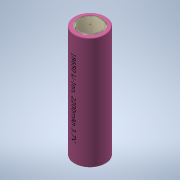
# Autodesk Inventor part: 18650
Saved by Autodesk Inventor 2022 (Build 260153070, 153G)
## iProperties
Created: 2016-01-10
Part Number: 18650
Material: Generic
Document SubType Name: Modeling
Designer: Kostic
Density: 1 g/cm^3
Appearance: Default
GlobalPropertyList: <PropertyList/>
Author: Kostic
Autodesk Inventor part; units mm, degrees
ref_plane "YZ Plane" through (0, 0, 0) normal (1, 0, 0) x (0, 1, 0)
ref_plane "XY Plane" through (0, 0, 0) normal (0, 0, 1) x (1, 0, 0)
sketch "Sketch1" plane through (0, 0, 0) normal (0, 0, 1) x (1, 0, 0)
  circle A0 centre (0, 0) radius 9
  dimension "d0" = 18
  constraints: 1 centre point, 1 coincident
  measures "d0" diameter of A0
extrude "Extrusion1" add sketch "Sketch1" along normal blind 64.7
sketch "Sketch2" plane through (0, 0, 64.7) normal (0, 0, 1) x (1, 0, 0)
  circle A0 centre (0, 0) radius 6
  dimension "d3" = 12
  constraints: 1 centre point, 1 coincident
  measures "d3" diameter of A0
extrude "Extrusion2" add sketch "Sketch2" along normal blind 0.1
sketch "Sketch3" plane through (0, 0, 0) normal (0, 0, -1) x (-1, 0, 0)
  circle A0 centre (0, 0) radius 7
  dimension "d6" = 14
  constraints: 1 centre point, 1 coincident
  measures "d6" diameter of A0
extrude "Extrusion3" cut sketch "Sketch3" against normal blind 0.1
fillet "Fillet1" radius 0.5 2 edges at (-9, 0, 64.7) (-9, 0, 0)
sketch "Sketch4" plane through (0, 0, 64.7) normal (0, 0, 1) x (1, 0, 0)
  circle A0 centre (0, 0) radius 7
  circle A1 centre (0, 0) radius 6
  dimension "d10" = 14
  dimension "d11" = 12
  constraints: 2 centre point, 2 coincident
  measures "d10" diameter of A0
  measures "d11" diameter of A1
extrude "Extrusion4" cut sketch "Sketch4" against normal blind 0.6
fillet "Fillet2" radius 0.5 2 edges at (-7, 0, 64.1) (-6, 0, 64.1)
fillet "Fillet3" radius 0.1 1 edges at (-6, 0, 64.8)
ref_plane "Work Plane1" through (0, -9, 0) normal (0, -1, 0) x (1, 0, 0)
sketch "Sketch5" plane through (0, -9, 0) normal (0, -1, 0) x (1, 0, 0)
  line L0 (0.9968, 55) -> (0.9968, -8.1341) construction
  line L1 (0.9968, -8.1341) -> (-3.5299, -8.1341) construction
  line L2 (-3.5299, -8.1341) -> (-3.5299, 55) construction
  line L3 (-3.5299, 55) -> (0.9968, 55) construction
  line L4 (8.5, 0) -> (-8.5, 0) projected
  line L5 (-1.6564, 53.376) -> (-1.6564, 54.6151)
  line L6 (-1.6564, 54.6151) -> (-1.397, 54.6151)
  line L7 (-1.397, 54.6151) -> (-1.397, 54.154)
  line L8 (-1.397, 54.154) -> (0.3052, 54.154)
  line L9 (0.3052, 54.154) -> (0.3052, 54.6151)
  line L10 (0.3052, 54.6151) -> (0.5378, 54.6151)
  spline S0 degree 2 poles (0.5378, 54.6151) (0.5378, 54.3537) (0.686, 54.1067) (0.8919, 54.0902) knots 0 0 0 1 2 2 2
  line L11 (0.8919, 54.0902) -> (0.8919, 53.8267)
  line L12 (0.8919, 53.8267) -> (-1.397, 53.8267)
  line L13 (-1.397, 53.8267) -> (-1.397, 53.376)
  line L14 (-1.397, 53.376) -> (-1.6564, 53.376)
  spline S1 degree 2 poles (-1.714, 52.141) (-1.714, 52.3303) (-1.6008, 52.6411) (-1.4958, 52.7502) knots 0 0 0 1 2 2 2
  spline S2 degree 2 poles (-1.4958, 52.7502) (-1.3929, 52.8573) (-1.113, 52.9684) (-0.9545, 52.9684) knots 0 0 0 1 2 2 2
  spline S3 degree 2 poles (-0.9545, 52.9684) (-0.7486, 52.9684) (-0.4028, 52.7482) (-0.2999, 52.5382) knots 0 0 0 1 2 2 2
  line L15 (-0.2999, 52.5382) -> (-0.2896, 52.5382)
  spline S4 degree 2 poles (-0.2896, 52.5382) (-0.1805, 52.7255) (0.0788, 52.9067) (0.2723, 52.9067) knots 0 0 0 1 2 2 2
  spline S5 degree 2 poles (0.2723, 52.9067) (0.5584, 52.9067) (0.9413, 52.4744) (0.9413, 52.141) knots 0 0 0 1 2 2 2
  spline S6 degree 2 poles (0.9413, 52.141) (0.9413, 51.7952) (0.579, 51.3773) (0.295, 51.3773) knots 0 0 0 1 2 2 2
  spline S7 degree 2 poles (0.295, 51.3773) (0.1241, 51.3773) (-0.2093, 51.577) (-0.304, 51.7643) knots 0 0 0 1 2 2 2
  line L16 (-0.304, 51.7643) -> (-0.3143, 51.7643)
  spline S8 degree 2 poles (-0.3143, 51.7643) (-0.4172, 51.542) (-0.7136, 51.3135) (-0.9483, 51.3135) knots 0 0 0 1 2 2 2
  spline S9 degree 2 poles (-0.9483, 51.3135) (-1.2735, 51.3135) (-1.714, 51.7869) (-1.714, 52.141) knots 0 0 0 1 2 2 2
  spline S10 degree 2 poles (-0.9812, 51.6634) (-0.8248, 51.6634) (-0.6395, 51.7869) (-0.5449, 51.9619) knots 0 0 0 1 2 2 2
  spline S11 degree 2 poles (-0.5449, 51.9619) (-0.5119, 52.0195) (-0.4358, 52.213) (-0.3864, 52.3344) knots 0 0 0 1 2 2 2
  spline S12 degree 2 poles (-0.3864, 52.3344) (-0.479, 52.4744) (-0.7548, 52.6247) (-0.9298, 52.6247) knots 0 0 0 1 2 2 2
  spline S13 degree 2 poles (-0.9298, 52.6247) (-1.1603, 52.6247) (-1.4608, 52.3468) (-1.4608, 52.1368) knots 0 0 0 1 2 2 2
  spline S14 degree 2 poles (-1.4608, 52.1368) (-1.4608, 51.9228) (-1.2035, 51.6634) (-0.9812, 51.6634) knots 0 0 0 1 2 2 2
  spline S15 degree 2 poles (0.2908, 51.7108) (0.4617, 51.7108) (0.6902, 51.9392) (0.6902, 52.143) knots 0 0 0 1 2 2 2
  spline S16 degree 2 poles (0.6902, 52.143) (0.6902, 52.3283) (0.4864, 52.565) (0.3114, 52.565) knots 0 0 0 1 2 2 2
  spline S17 degree 2 poles (0.3114, 52.565) (0.1859, 52.565) (0.0109, 52.4435) (-0.0591, 52.3221) knots 0 0 0 1 2 2 2
  spline S18 degree 2 poles (-0.0591, 52.3221) (-0.0879, 52.2706) (-0.1888, 52.0524) (-0.2176, 51.9639) knots 0 0 0 1 2 2 2
  spline S19 degree 2 poles (-0.2176, 51.9639) (-0.1044, 51.8157) (0.1365, 51.7108) (0.2908, 51.7108) knots 0 0 0 1 2 2 2
  spline S20 degree 2 poles (-0.833, 49.3972) (-1.0286, 49.3972) (-1.36, 49.5269) (-1.4711, 49.6359) knots 0 0 0 1 2 2 2
  spline S21 degree 2 poles (-1.4711, 49.6359) (-1.5884, 49.7492) (-1.7099, 50.0332) (-1.7099, 50.2041) knots 0 0 0 1 2 2 2
  spline S22 degree 2 poles (-1.7099, 50.2041) (-1.7099, 50.3749) (-1.5946, 50.6569) (-1.4793, 50.7639) knots 0 0 0 1 2 2 2
  spline S23 degree 2 poles (-1.4793, 50.7639) (-1.3414, 50.8957) (-0.8783, 51.0439) (-0.5407, 51.0439) knots 0 0 0 1 2 2 2
  spline S24 degree 2 poles (-0.5407, 51.0439) (-0.2093, 51.0439) (0.3238, 50.908) (0.5214, 50.766) knots 0 0 0 1 2 2 2
  spline S25 degree 2 poles (0.5214, 50.766) (0.7149, 50.6281) (0.931, 50.1917) (0.931, 49.9056) knots 0 0 0 1 2 2 2
  spline S26 degree 2 poles (0.931, 49.9056) (0.931, 49.8212) (0.9145, 49.673) (0.896, 49.6174) knots 0 0 0 1 2 2 2
  line L17 (0.896, 49.6174) -> (0.5687, 49.6174)
  line L18 (0.5687, 49.6174) -> (0.5687, 49.6318)
  spline S27 degree 2 poles (0.5687, 49.6318) (0.5934, 49.6792) (0.6366, 49.8521) (0.6366, 49.9509) knots 0 0 0 1 2 2 2
  spline S28 degree 2 poles (0.6366, 49.9509) (0.6366, 50.2679) (0.2085, 50.6569) (-0.2114, 50.6939) knots 0 0 0 1 2 2 2
  spline S29 degree 2 poles (-0.2114, 50.6939) (-0.127, 50.5725) (-0.0344, 50.3173) (-0.0344, 50.1649) knots 0 0 0 1 2 2 2
  spline S30 degree 2 poles (-0.0344, 50.1649) (-0.0344, 50.0167) (-0.0941, 49.7944) (-0.1846, 49.673) knots 0 0 0 1 2 2 2
  spline S31 degree 2 poles (-0.1846, 49.673) (-0.2896, 49.533) (-0.6148, 49.3972) (-0.833, 49.3972) knots 0 0 0 1 2 2 2
  spline S32 degree 2 poles (-0.8474, 49.743) (-0.691, 49.743) (-0.479, 49.8253) (-0.4049, 49.9159) knots 0 0 0 1 2 2 2
  spline S33 degree 2 poles (-0.4049, 49.9159) (-0.3514, 49.9838) (-0.3164, 50.1526) (-0.3164, 50.2411) knots 0 0 0 1 2 2 2
  spline S34 degree 2 poles (-0.3164, 50.2411) (-0.3164, 50.3605) (-0.3884, 50.5848) (-0.4563, 50.6939) knots 0 0 0 1 2 2 2
  spline S35 degree 2 poles (-0.4563, 50.6939) (-0.4934, 50.696) (-0.5634, 50.7001) (-0.6169, 50.7001) knots 0 0 0 1 2 2 2
  spline S36 degree 2 poles (-0.6169, 50.7001) (-0.8804, 50.7001) (-1.2035, 50.5972) (-1.2879, 50.519) knots 0 0 0 1 2 2 2
  spline S37 degree 2 poles (-1.2879, 50.519) (-1.3682, 50.4469) (-1.432, 50.2905) (-1.432, 50.202) knots 0 0 0 1 2 2 2
  spline S38 degree 2 poles (-1.432, 50.202) (-1.432, 49.9962) (-1.1397, 49.743) (-0.8474, 49.743) knots 0 0 0 1 2 2 2
  spline S39 degree 2 poles (-0.8495, 47.557) (-1.0327, 47.557) (-1.3455, 47.6743) (-1.4608, 47.7814) knots 0 0 0 1 2 2 2
  spline S40 degree 2 poles (-1.4608, 47.7814) (-1.5761, 47.8884) (-1.7099, 48.2075) (-1.7099, 48.4051) knots 0 0 0 1 2 2 2
  spline S41 degree 2 poles (-1.7099, 48.4051) (-1.7099, 48.5862) (-1.6296, 48.9402) (-1.5658, 49.0699) knots 0 0 0 1 2 2 2
  line L19 (-1.5658, 49.0699) -> (-1.2056, 49.0699)
  line L20 (-1.2056, 49.0699) -> (-1.2056, 49.0452)
  spline S42 degree 2 poles (-1.2056, 49.0452) (-1.2344, 49.0061) (-1.3085, 48.86) (-1.3414, 48.7714) knots 0 0 0 1 2 2 2
  spline S43 degree 2 poles (-1.3414, 48.7714) (-1.3764, 48.6706) (-1.4155, 48.5039) (-1.4155, 48.3989) knots 0 0 0 1 2 2 2
  spline S44 degree 2 poles (-1.4155, 48.3989) (-1.4155, 48.296) (-1.3414, 48.1025) (-1.2612, 48.0325) knots 0 0 0 1 2 2 2
  spline S45 degree 2 poles (-1.2612, 48.0325) (-1.185, 47.9687) (-0.9833, 47.9028) (-0.8474, 47.9028) knots 0 0 0 1 2 2 2
  spline S46 degree 2 poles (-0.8474, 47.9028) (-0.7116, 47.9028) (-0.5387, 47.9769) (-0.481, 48.0469) knots 0 0 0 1 2 2 2
  spline S47 degree 2 poles (-0.481, 48.0469) (-0.4172, 48.1189) (-0.3637, 48.333) (-0.3637, 48.4627) knots 0 0 0 1 2 2 2
  spline S48 degree 2 poles (-0.3637, 48.4627) (-0.3637, 48.6027) (-0.4069, 48.8805) (-0.4255, 48.9649) knots 0 0 0 1 2 2 2
  line L21 (-0.4255, 48.9649) -> (0.8836, 48.9649)
  line L22 (0.8836, 48.9649) -> (0.8836, 47.5714)
  line L23 (0.8836, 47.5714) -> (0.5852, 47.5714)
  line L24 (0.5852, 47.5714) -> (0.5852, 48.6376)
  line L25 (0.5852, 48.6376) -> (-0.092, 48.6376)
  spline S49 degree 2 poles (-0.092, 48.6376) (-0.0838, 48.5759) (-0.0776, 48.4565) (-0.0776, 48.4071) knots 0 0 0 1 2 2 2
  spline S50 degree 2 poles (-0.0776, 48.4071) (-0.0776, 48.2116) (-0.1414, 47.9419) (-0.2361, 47.8184) knots 0 0 0 1 2 2 2
  spline S51 degree 2 poles (-0.2361, 47.8184) (-0.3308, 47.6929) (-0.619, 47.557) (-0.8495, 47.557) knots 0 0 0 1 2 2 2
  spline S52 degree 2 poles (-0.3864, 45.6098) (-1.0697, 45.6098) (-1.7099, 46.0071) (-1.7099, 46.4208) knots 0 0 0 1 2 2 2
  spline S53 degree 2 poles (-1.7099, 46.4208) (-1.7099, 46.8407) (-1.0574, 47.2339) (-0.3884, 47.2339) knots 0 0 0 1 2 2 2
  spline S54 degree 2 poles (-0.3884, 47.2339) (0.2991, 47.2339) (0.9351, 46.8366) (0.9351, 46.4208) knots 0 0 0 1 2 2 2
  spline S55 degree 2 poles (0.9351, 46.4208) (0.9351, 46.003) (0.2764, 45.6098) (-0.3864, 45.6098) knots 0 0 0 1 2 2 2
  spline S56 degree 2 poles (-1.1603, 46.0462) (-1.0347, 45.9968) (-0.6478, 45.9556) (-0.3864, 45.9556) knots 0 0 0 1 2 2 2
  spline S57 degree 2 poles (-0.3864, 45.9556) (-0.1249, 45.9556) (0.26, 45.9968) (0.3896, 46.0482) knots 0 0 0 1 2 2 2
  spline S58 degree 2 poles (0.3896, 46.0482) (0.5193, 46.0997) (0.6531, 46.2788) (0.6531, 46.4208) knots 0 0 0 1 2 2 2
  spline S59 degree 2 poles (0.6531, 46.4208) (0.6531, 46.5628) (0.5193, 46.746) (0.3855, 46.7995) knots 0 0 0 1 2 2 2
  spline S60 degree 2 poles (0.3855, 46.7995) (0.2558, 46.851) (-0.1394, 46.8881) (-0.3884, 46.8881) knots 0 0 0 1 2 2 2
  spline S61 degree 2 poles (-0.3884, 46.8881) (-0.656, 46.8881) (-1.0142, 46.8551) (-1.1541, 46.8016) knots 0 0 0 1 2 2 2
  spline S62 degree 2 poles (-1.1541, 46.8016) (-1.2859, 46.7522) (-1.4279, 46.569) (-1.4279, 46.4208) knots 0 0 0 1 2 2 2
  spline S63 degree 2 poles (-1.4279, 46.4208) (-1.4279, 46.2808) (-1.2941, 46.0976) (-1.1603, 46.0462) knots 0 0 0 1 2 2 2
  line L26 (-1.6564, 42.6499) -> (-1.6564, 44.1216)
  line L27 (-1.6564, 44.1216) -> (0.8836, 44.1216)
  line L28 (0.8836, 44.1216) -> (0.8836, 43.7841)
  line L29 (0.8836, 43.7841) -> (-1.3558, 43.7841)
  line L30 (-1.3558, 43.7841) -> (-1.3558, 42.6499)
  line L31 (-1.3558, 42.6499) -> (-1.6564, 42.6499)
  line L32 (-1.6564, 42.0818) -> (-1.6564, 42.4029)
  line L33 (-1.6564, 42.4029) -> (0.2497, 42.4029)
  line L34 (0.2497, 42.4029) -> (0.2497, 42.0818)
  line L35 (0.2497, 42.0818) -> (-1.6564, 42.0818)
  line L36 (0.5667, 42.0592) -> (0.5667, 42.4235)
  line L37 (0.5667, 42.4235) -> (0.9001, 42.4235)
  line L38 (0.9001, 42.4235) -> (0.9001, 42.0592)
  line L39 (0.9001, 42.0592) -> (0.5667, 42.0592)
  line L40 (-0.6992, 40.7274) -> (-0.6992, 41.6887)
  line L41 (-0.6992, 41.6887) -> (-0.3905, 41.6887)
  line L42 (-0.3905, 41.6887) -> (-0.3905, 40.7274)
  line L43 (-0.3905, 40.7274) -> (-0.6992, 40.7274)
  line L44 (-1.6564, 39.4327) -> (-1.6564, 40.4166)
  line L45 (-1.6564, 40.4166) -> (-1.397, 40.4166)
  line L46 (-1.397, 40.4166) -> (-1.397, 40.0935)
  line L47 (-1.397, 40.0935) -> (0.6243, 40.0935)
  line L48 (0.6243, 40.0935) -> (0.6243, 40.4166)
  line L49 (0.6243, 40.4166) -> (0.8836, 40.4166)
  line L50 (0.8836, 40.4166) -> (0.8836, 39.4327)
  line L51 (0.8836, 39.4327) -> (0.6243, 39.4327)
  line L52 (0.6243, 39.4327) -> (0.6243, 39.7559)
  line L53 (0.6243, 39.7559) -> (-1.397, 39.7559)
  line L54 (-1.397, 39.7559) -> (-1.397, 39.4327)
  line L55 (-1.397, 39.4327) -> (-1.6564, 39.4327)
  spline S64 degree 2 poles (-0.7033, 37.4732) (-1.185, 37.4732) (-1.7099, 37.9363) (-1.7099, 38.3233) knots 0 0 0 1 2 2 2
  spline S65 degree 2 poles (-1.7099, 38.3233) (-1.7099, 38.7205) (-1.1685, 39.1754) (-0.7033, 39.1754) knots 0 0 0 1 2 2 2
  spline S66 degree 2 poles (-0.7033, 39.1754) (-0.2258, 39.1754) (0.3032, 38.7061) (0.3032, 38.3233) knots 0 0 0 1 2 2 2
  spline S67 degree 2 poles (0.3032, 38.3233) (0.3032, 37.9363) (-0.2238, 37.4732) (-0.7033, 37.4732) knots 0 0 0 1 2 2 2
  spline S68 degree 2 poles (-0.7033, 37.8046) (-0.3328, 37.8046) (0.0274, 38.0742) (0.0274, 38.3233) knots 0 0 0 1 2 2 2
  spline S69 degree 2 poles (0.0274, 38.3233) (0.0274, 38.5723) (-0.3328, 38.844) (-0.7033, 38.844) knots 0 0 0 1 2 2 2
  spline S70 degree 2 poles (-0.7033, 38.844) (-1.0636, 38.844) (-1.4341, 38.5723) (-1.4341, 38.3233) knots 0 0 0 1 2 2 2
  spline S71 degree 2 poles (-1.4341, 38.3233) (-1.4341, 38.0763) (-1.0697, 37.8046) (-0.7033, 37.8046) knots 0 0 0 1 2 2 2
  line L56 (-1.6564, 35.6474) -> (-1.6564, 35.9685)
  line L57 (-1.6564, 35.9685) -> (-0.5696, 35.9685)
  spline S72 degree 2 poles (-0.5696, 35.9685) (-0.4378, 35.9685) (-0.2114, 35.9932) (-0.1435, 36.0303) knots 0 0 0 1 2 2 2
  spline S73 degree 2 poles (-0.1435, 36.0303) (-0.0714, 36.0694) (-0.0014, 36.2094) (-0.0014, 36.3287) knots 0 0 0 1 2 2 2
  spline S74 degree 2 poles (-0.0014, 36.3287) (-0.0014, 36.4481) (-0.1291, 36.7013) (-0.232, 36.8227) knots 0 0 0 1 2 2 2
  line L58 (-0.232, 36.8227) -> (-1.6564, 36.8227)
  line L59 (-1.6564, 36.8227) -> (-1.6564, 37.1438)
  line L60 (-1.6564, 37.1438) -> (0.2497, 37.1438)
  line L61 (0.2497, 37.1438) -> (0.2497, 36.8227)
  line L62 (0.2497, 36.8227) -> (0.0377, 36.8227)
  spline S75 degree 2 poles (0.0377, 36.8227) (0.1673, 36.6787) (0.3032, 36.4008) (0.3032, 36.2443) knots 0 0 0 1 2 2 2
  spline S76 degree 2 poles (0.3032, 36.2443) (0.3032, 35.9644) (-0.0673, 35.6474) (-0.4193, 35.6474) knots 0 0 0 1 2 2 2
  line L63 (-0.4193, 35.6474) -> (-1.6564, 35.6474)
  line L64 (-1.1706, 34.5771) -> (-2.2883, 35.0546)
  line L65 (-2.2883, 35.0546) -> (-2.2883, 35.3037)
  line L66 (-2.2883, 35.3037) -> (-1.1706, 35.0032)
  line L67 (-1.1706, 35.0032) -> (-1.1706, 34.5771)
  line L68 (-1.6564, 31.5287) -> (-1.6564, 33.0951)
  line L69 (-1.6564, 33.0951) -> (-1.2961, 33.0951)
  spline S77 degree 2 poles (-1.2961, 33.0951) (-1.1377, 32.9263) (-0.8433, 32.6258) (-0.6848, 32.4817) knots 0 0 0 1 2 2 2
  spline S78 degree 2 poles (-0.6848, 32.4817) (-0.3658, 32.1915) (0.0171, 31.9794) (0.2209, 31.9794) knots 0 0 0 1 2 2 2
  spline S79 degree 2 poles (0.2209, 31.9794) (0.3279, 31.9794) (0.4884, 32.0453) (0.5399, 32.105) knots 0 0 0 1 2 2 2
  spline S80 degree 2 poles (0.5399, 32.105) (0.5914, 32.1647) (0.6428, 32.3211) (0.6428, 32.4158) knots 0 0 0 1 2 2 2
  spline S81 degree 2 poles (0.6428, 32.4158) (0.6428, 32.5064) (0.5975, 32.6916) (0.5625, 32.776) knots 0 0 0 1 2 2 2
  spline S82 degree 2 poles (0.5625, 32.776) (0.5337, 32.8481) (0.4514, 32.9819) (0.4226, 33.023) knots 0 0 0 1 2 2 2
  line L70 (0.4226, 33.023) -> (0.4226, 33.0416)
  line L71 (0.4226, 33.0416) -> (0.7848, 33.0416)
  spline S83 degree 2 poles (0.7848, 33.0416) (0.8363, 32.9366) (0.9372, 32.5599) (0.9372, 32.3911) knots 0 0 0 1 2 2 2
  spline S84 degree 2 poles (0.9372, 32.3911) (0.9372, 32.035) (0.5605, 31.6336) (0.2394, 31.6336) knots 0 0 0 1 2 2 2
  spline S85 degree 2 poles (0.2394, 31.6336) (0.0891, 31.6336) (-0.162, 31.7036) (-0.269, 31.7654) knots 0 0 0 1 2 2 2
  spline S86 degree 2 poles (-0.269, 31.7654) (-0.3802, 31.8271) (-0.5984, 32.0062) (-0.7033, 32.105) knots 0 0 0 1 2 2 2
  spline S87 degree 2 poles (-0.7033, 32.105) (-0.8783, 32.2656) (-1.2529, 32.6587) (-1.362, 32.776) knots 0 0 0 1 2 2 2
  line L72 (-1.362, 32.776) -> (-1.362, 31.5287)
  line L73 (-1.362, 31.5287) -> (-1.6564, 31.5287)
  line L74 (-1.6564, 29.6226) -> (-1.6564, 31.189)
  line L75 (-1.6564, 31.189) -> (-1.2961, 31.189)
  spline S88 degree 2 poles (-1.2961, 31.189) (-1.1377, 31.0203) (-0.8433, 30.7197) (-0.6848, 30.5757) knots 0 0 0 1 2 2 2
  spline S89 degree 2 poles (-0.6848, 30.5757) (-0.3658, 30.2854) (0.0171, 30.0734) (0.2209, 30.0734) knots 0 0 0 1 2 2 2
  spline S90 degree 2 poles (0.2209, 30.0734) (0.3279, 30.0734) (0.4884, 30.1393) (0.5399, 30.199) knots 0 0 0 1 2 2 2
  spline S91 degree 2 poles (0.5399, 30.199) (0.5914, 30.2587) (0.6428, 30.4151) (0.6428, 30.5098) knots 0 0 0 1 2 2 2
  spline S92 degree 2 poles (0.6428, 30.5098) (0.6428, 30.6004) (0.5975, 30.7856) (0.5625, 30.87) knots 0 0 0 1 2 2 2
  spline S93 degree 2 poles (0.5625, 30.87) (0.5337, 30.942) (0.4514, 31.0758) (0.4226, 31.117) knots 0 0 0 1 2 2 2
  line L76 (0.4226, 31.117) -> (0.4226, 31.1355)
  line L77 (0.4226, 31.1355) -> (0.7848, 31.1355)
  spline S94 degree 2 poles (0.7848, 31.1355) (0.8363, 31.0306) (0.9372, 30.6539) (0.9372, 30.4851) knots 0 0 0 1 2 2 2
  spline S95 degree 2 poles (0.9372, 30.4851) (0.9372, 30.129) (0.5605, 29.7276) (0.2394, 29.7276) knots 0 0 0 1 2 2 2
  spline S96 degree 2 poles (0.2394, 29.7276) (0.0891, 29.7276) (-0.162, 29.7976) (-0.269, 29.8594) knots 0 0 0 1 2 2 2
  spline S97 degree 2 poles (-0.269, 29.8594) (-0.3802, 29.9211) (-0.5984, 30.1002) (-0.7033, 30.199) knots 0 0 0 1 2 2 2
  spline S98 degree 2 poles (-0.7033, 30.199) (-0.8783, 30.3595) (-1.2529, 30.7527) (-1.362, 30.87) knots 0 0 0 1 2 2 2
  line L78 (-1.362, 30.87) -> (-1.362, 29.6226)
  line L79 (-1.362, 29.6226) -> (-1.6564, 29.6226)
  spline S99 degree 2 poles (-0.3864, 27.7022) (-1.0697, 27.7022) (-1.7099, 28.0995) (-1.7099, 28.5132) knots 0 0 0 1 2 2 2
  spline S100 degree 2 poles (-1.7099, 28.5132) (-1.7099, 28.9331) (-1.0574, 29.3262) (-0.3884, 29.3262) knots 0 0 0 1 2 2 2
  spline S101 degree 2 poles (-0.3884, 29.3262) (0.2991, 29.3262) (0.9351, 28.929) (0.9351, 28.5132) knots 0 0 0 1 2 2 2
  spline S102 degree 2 poles (0.9351, 28.5132) (0.9351, 28.0953) (0.2764, 27.7022) (-0.3864, 27.7022) knots 0 0 0 1 2 2 2
  spline S103 degree 2 poles (-1.1603, 28.1386) (-1.0347, 28.0892) (-0.6478, 28.048) (-0.3864, 28.048) knots 0 0 0 1 2 2 2
  spline S104 degree 2 poles (-0.3864, 28.048) (-0.1249, 28.048) (0.26, 28.0892) (0.3896, 28.1406) knots 0 0 0 1 2 2 2
  spline S105 degree 2 poles (0.3896, 28.1406) (0.5193, 28.1921) (0.6531, 28.3712) (0.6531, 28.5132) knots 0 0 0 1 2 2 2
  spline S106 degree 2 poles (0.6531, 28.5132) (0.6531, 28.6552) (0.5193, 28.8384) (0.3855, 28.8919) knots 0 0 0 1 2 2 2
  spline S107 degree 2 poles (0.3855, 28.8919) (0.2558, 28.9434) (-0.1394, 28.9804) (-0.3884, 28.9804) knots 0 0 0 1 2 2 2
  spline S108 degree 2 poles (-0.3884, 28.9804) (-0.656, 28.9804) (-1.0142, 28.9475) (-1.1541, 28.894) knots 0 0 0 1 2 2 2
  spline S109 degree 2 poles (-1.1541, 28.894) (-1.2859, 28.8446) (-1.4279, 28.6614) (-1.4279, 28.5132) knots 0 0 0 1 2 2 2
  spline S110 degree 2 poles (-1.4279, 28.5132) (-1.4279, 28.3732) (-1.2941, 28.19) (-1.1603, 28.1386) knots 0 0 0 1 2 2 2
  spline S111 degree 2 poles (-0.3864, 25.7962) (-1.0697, 25.7962) (-1.7099, 26.1934) (-1.7099, 26.6072) knots 0 0 0 1 2 2 2
  spline S112 degree 2 poles (-1.7099, 26.6072) (-1.7099, 27.0271) (-1.0574, 27.4202) (-0.3884, 27.4202) knots 0 0 0 1 2 2 2
  spline S113 degree 2 poles (-0.3884, 27.4202) (0.2991, 27.4202) (0.9351, 27.0229) (0.9351, 26.6072) knots 0 0 0 1 2 2 2
  spline S114 degree 2 poles (0.9351, 26.6072) (0.9351, 26.1893) (0.2764, 25.7962) (-0.3864, 25.7962) knots 0 0 0 1 2 2 2
  spline S115 degree 2 poles (-1.1603, 26.2325) (-1.0347, 26.1831) (-0.6478, 26.142) (-0.3864, 26.142) knots 0 0 0 1 2 2 2
  spline S116 degree 2 poles (-0.3864, 26.142) (-0.1249, 26.142) (0.26, 26.1831) (0.3896, 26.2346) knots 0 0 0 1 2 2 2
  spline S117 degree 2 poles (0.3896, 26.2346) (0.5193, 26.2861) (0.6531, 26.4651) (0.6531, 26.6072) knots 0 0 0 1 2 2 2
  spline S118 degree 2 poles (0.6531, 26.6072) (0.6531, 26.7492) (0.5193, 26.9324) (0.3855, 26.9859) knots 0 0 0 1 2 2 2
  spline S119 degree 2 poles (0.3855, 26.9859) (0.2558, 27.0374) (-0.1394, 27.0744) (-0.3884, 27.0744) knots 0 0 0 1 2 2 2
  spline S120 degree 2 poles (-0.3884, 27.0744) (-0.656, 27.0744) (-1.0142, 27.0415) (-1.1541, 26.988) knots 0 0 0 1 2 2 2
  spline S121 degree 2 poles (-1.1541, 26.988) (-1.2859, 26.9386) (-1.4279, 26.7554) (-1.4279, 26.6072) knots 0 0 0 1 2 2 2
  spline S122 degree 2 poles (-1.4279, 26.6072) (-1.4279, 26.4672) (-1.2941, 26.284) (-1.1603, 26.2325) knots 0 0 0 1 2 2 2
  line L80 (-1.6564, 23.2623) -> (-0.5531, 23.2623)
  spline S123 degree 2 poles (-0.5531, 23.2623) (-0.4214, 23.2623) (-0.197, 23.2829) (-0.1352, 23.3159) knots 0 0 0 1 2 2 2
  spline S124 degree 2 poles (-0.1352, 23.3159) (-0.0673, 23.3488) (-0.0014, 23.4744) (-0.0014, 23.5835) knots 0 0 0 1 2 2 2
  spline S125 degree 2 poles (-0.0014, 23.5835) (-0.0014, 23.6823) (-0.1229, 23.9087) (-0.2382, 24.0281) knots 0 0 0 1 2 2 2
  spline S126 degree 2 poles (-0.2382, 24.0281) (-0.267, 24.026) (-0.3473, 24.0219) (-0.4008, 24.0219) knots 0 0 0 1 2 2 2
  line L81 (-0.4008, 24.0219) -> (-1.6564, 24.0219)
  line L82 (-1.6564, 24.0219) -> (-1.6564, 24.343)
  line L83 (-1.6564, 24.343) -> (-0.5531, 24.343)
  spline S127 degree 2 poles (-0.5531, 24.343) (-0.4214, 24.343) (-0.197, 24.3636) (-0.1352, 24.3965) knots 0 0 0 1 2 2 2
  spline S128 degree 2 poles (-0.1352, 24.3965) (-0.0673, 24.4294) (-0.0014, 24.555) (-0.0014, 24.6641) knots 0 0 0 1 2 2 2
  spline S129 degree 2 poles (-0.0014, 24.6641) (-0.0014, 24.767) (-0.1311, 24.9955) (-0.232, 25.1025) knots 0 0 0 1 2 2 2
  line L84 (-0.232, 25.1025) -> (-1.6564, 25.1025)
  line L85 (-1.6564, 25.1025) -> (-1.6564, 25.4236)
  line L86 (-1.6564, 25.4236) -> (0.2497, 25.4236)
  line L87 (0.2497, 25.4236) -> (0.2497, 25.1025)
  line L88 (0.2497, 25.1025) -> (0.0397, 25.1025)
  spline S130 degree 2 poles (0.0397, 25.1025) (0.1653, 24.977) (0.3032, 24.73) (0.3032, 24.5817) knots 0 0 0 1 2 2 2
  spline S131 degree 2 poles (0.3032, 24.5817) (0.3032, 24.413) (0.1488, 24.1516) (-0.0261, 24.0836) knots 0 0 0 1 2 2 2
  spline S132 degree 2 poles (-0.0261, 24.0836) (0.1365, 23.9375) (0.3032, 23.6617) (0.3032, 23.5011) knots 0 0 0 1 2 2 2
  spline S133 degree 2 poles (0.3032, 23.5011) (0.3032, 23.3776) (0.227, 23.1759) (0.1406, 23.1018) knots 0 0 0 1 2 2 2
  spline S134 degree 2 poles (0.1406, 23.1018) (0.0541, 23.0256) (-0.2052, 22.9412) (-0.4008, 22.9412) knots 0 0 0 1 2 2 2
  line L89 (-0.4008, 22.9412) -> (-1.6564, 22.9412)
  line L90 (-1.6564, 22.9412) -> (-1.6564, 23.2623)
  line L91 (-1.6564, 22.7395) -> (0.8836, 21.8833)
  line L92 (0.8836, 21.8833) -> (0.8836, 21.4675)
  line L93 (0.8836, 21.4675) -> (-1.6564, 20.6112)
  line L94 (-1.6564, 20.6112) -> (-1.6564, 20.9673)
  line L95 (-1.6564, 20.9673) -> (-0.9462, 21.1978)
  line L96 (-0.9462, 21.1978) -> (-0.9462, 22.1673)
  line L97 (-0.9462, 22.1673) -> (-1.6564, 22.3978)
  line L98 (-1.6564, 22.3978) -> (-1.6564, 22.7395)
  line L99 (-0.6581, 21.2905) -> (0.5378, 21.6836)
  line L100 (0.5378, 21.6836) -> (-0.6581, 22.0747)
  line L101 (-0.6581, 22.0747) -> (-0.6581, 21.2905)
  line L102 (-1.6564, 18.8987) -> (-1.6564, 19.2198)
  line L103 (-1.6564, 19.2198) -> (-0.5696, 19.2198)
  spline S135 degree 2 poles (-0.5696, 19.2198) (-0.4378, 19.2198) (-0.2114, 19.2445) (-0.1435, 19.2815) knots 0 0 0 1 2 2 2
  spline S136 degree 2 poles (-0.1435, 19.2815) (-0.0714, 19.3206) (-0.0014, 19.4606) (-0.0014, 19.58) knots 0 0 0 1 2 2 2
  spline S137 degree 2 poles (-0.0014, 19.58) (-0.0014, 19.6994) (-0.1291, 19.9525) (-0.232, 20.074) knots 0 0 0 1 2 2 2
  line L104 (-0.232, 20.074) -> (-1.6564, 20.074)
  line L105 (-1.6564, 20.074) -> (-1.6564, 20.3951)
  line L106 (-1.6564, 20.3951) -> (0.9968, 20.3951)
  line L107 (0.9968, 20.3951) -> (0.9968, 20.074)
  line L108 (0.9968, 20.074) -> (0.0377, 20.074)
  spline S138 degree 2 poles (0.0377, 20.074) (0.1673, 19.9299) (0.3032, 19.652) (0.3032, 19.4956) knots 0 0 0 1 2 2 2
  spline S139 degree 2 poles (0.3032, 19.4956) (0.3032, 19.2156) (-0.0673, 18.8987) (-0.4193, 18.8987) knots 0 0 0 1 2 2 2
  line L109 (-0.4193, 18.8987) -> (-1.6564, 18.8987)
  spline S140 degree 2 poles (0.6428, 16.7189) (0.6428, 16.8115) (0.5975, 16.9947) (0.5625, 17.0832) knots 0 0 0 1 2 2 2
  spline S141 degree 2 poles (0.5625, 17.0832) (0.5275, 17.1655) (0.4534, 17.287) (0.4205, 17.3343) knots 0 0 0 1 2 2 2
  line L110 (0.4205, 17.3343) -> (0.4205, 17.3549)
  line L111 (0.4205, 17.3549) -> (0.7807, 17.3549)
  spline S142 degree 2 poles (0.7807, 17.3549) (0.8404, 17.2437) (0.9372, 16.8629) (0.9372, 16.6921) knots 0 0 0 1 2 2 2
  spline S143 degree 2 poles (0.9372, 16.6921) (0.9372, 16.5192) (0.8672, 16.2619) (0.7931, 16.1569) knots 0 0 0 1 2 2 2
  spline S144 degree 2 poles (0.7931, 16.1569) (0.7128, 16.0458) (0.4802, 15.9305) (0.3238, 15.9305) knots 0 0 0 1 2 2 2
  spline S145 degree 2 poles (0.3238, 15.9305) (0.1138, 15.9305) (-0.2032, 16.2063) (-0.2443, 16.3998) knots 0 0 0 1 2 2 2
  line L112 (-0.2443, 16.3998) -> (-0.269, 16.3998)
  spline S146 degree 2 poles (-0.269, 16.3998) (-0.2855, 16.3195) (-0.3596, 16.1364) (-0.4337, 16.0581) knots 0 0 0 1 2 2 2
  spline S147 degree 2 poles (-0.4337, 16.0581) (-0.5057, 15.9799) (-0.7363, 15.8811) (-0.903, 15.8811) knots 0 0 0 1 2 2 2
  spline S148 degree 2 poles (-0.903, 15.8811) (-1.0738, 15.8811) (-1.3641, 15.9984) (-1.4752, 16.1055) knots 0 0 0 1 2 2 2
  spline S149 degree 2 poles (-1.4752, 16.1055) (-1.5905, 16.2166) (-1.7099, 16.5316) (-1.7099, 16.7312) knots 0 0 0 1 2 2 2
  spline S150 degree 2 poles (-1.7099, 16.7312) (-1.7099, 16.9226) (-1.6173, 17.2973) (-1.5534, 17.4249) knots 0 0 0 1 2 2 2
  line L113 (-1.5534, 17.4249) -> (-1.1932, 17.4249)
  line L114 (-1.1932, 17.4249) -> (-1.1932, 17.4002)
  spline S151 degree 2 poles (-1.1932, 17.4002) (-1.2714, 17.2931) (-1.4155, 16.9309) (-1.4155, 16.7518) knots 0 0 0 1 2 2 2
  spline S152 degree 2 poles (-1.4155, 16.7518) (-1.4155, 16.6468) (-1.3497, 16.4369) (-1.2735, 16.3669) knots 0 0 0 1 2 2 2
  spline S153 degree 2 poles (-1.2735, 16.3669) (-1.1973, 16.299) (-1.0162, 16.2269) (-0.8783, 16.2269) knots 0 0 0 1 2 2 2
  spline S154 degree 2 poles (-0.8783, 16.2269) (-0.7404, 16.2269) (-0.5613, 16.3072) (-0.5099, 16.3792) knots 0 0 0 1 2 2 2
  spline S155 degree 2 poles (-0.5099, 16.3792) (-0.4584, 16.4513) (-0.4193, 16.6468) (-0.4193, 16.7621) knots 0 0 0 1 2 2 2
  line L115 (-0.4193, 16.7621) -> (-0.4193, 16.9062)
  line L116 (-0.4193, 16.9062) -> (-0.1373, 16.9062)
  line L117 (-0.1373, 16.9062) -> (-0.1373, 16.793)
  spline S156 degree 2 poles (-0.1373, 16.793) (-0.1373, 16.5645) (0.0809, 16.2763) (0.2888, 16.2763) knots 0 0 0 1 2 2 2
  spline S157 degree 2 poles (0.2888, 16.2763) (0.3855, 16.2763) (0.5234, 16.3504) (0.5646, 16.4101) knots 0 0 0 1 2 2 2
  spline S158 degree 2 poles (0.5646, 16.4101) (0.6078, 16.4739) (0.6428, 16.6304) (0.6428, 16.7189) knots 0 0 0 1 2 2 2
  line L118 (-1.6564, 14.9528) -> (-1.6564, 15.3604)
  line L119 (-1.6564, 15.3604) -> (-1.1706, 15.3604)
  line L120 (-1.1706, 15.3604) -> (-1.1706, 14.9528)
  line L121 (-1.1706, 14.9528) -> (-1.6564, 14.9528)
  line L122 (0.5028, 12.8451) -> (-1.6564, 13.9442)
  line L123 (-1.6564, 13.9442) -> (-1.6564, 14.3065)
  line L124 (-1.6564, 14.3065) -> (0.5852, 13.1456)
  line L125 (0.5852, 13.1456) -> (0.5852, 14.4567)
  line L126 (0.5852, 14.4567) -> (0.8836, 14.4567)
  line L127 (0.8836, 14.4567) -> (0.8836, 12.8451)
  line L128 (0.8836, 12.8451) -> (0.5028, 12.8451)
  line L129 (0.8836, 10.62) -> (-1.6564, 11.4948)
  line L130 (-1.6564, 11.4948) -> (-1.6564, 11.8591)
  line L131 (-1.6564, 11.8591) -> (0.8836, 12.7339)
  line L132 (0.8836, 12.7339) -> (0.8836, 12.3716)
  line L133 (0.8836, 12.3716) -> (-1.2262, 11.6677)
  line L134 (-1.2262, 11.6677) -> (0.8836, 10.9637)
  line L135 (0.8836, 10.9637) -> (0.8836, 10.62)
  point P0 (0, 0)
  dimension "d17" = 55
  constraints: 2 other
  measures "d17" distance between parallel lines of L4 L3
emboss "Emboss1" sketch "Sketch5" operation cut depth 0.01 direction (0, 1, 0)
pattern_circular "Circular Pattern1" count 2 over 360 about axis through (0, 0, 0) along (0, 0, 1) of "Emboss1"
body "Solid1"
